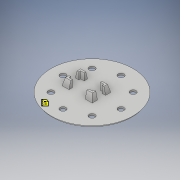
# Autodesk Inventor part: bottom_platform
Saved by Autodesk Inventor 2018 (Build 220112000, 112)
## iProperties
Created: 2018-04-16
Part Number: bottom_platform
Material: Generic
Document SubType Name: Modeling
Designer: scwu
Density: 1 g/cm^3
Appearance: Default
Author: scwu
Autodesk Inventor part; units mm, degrees
sketch "Sketch1" plane through (0, 0, 0) normal (0, 0, 1) x (1, 0, 0)
  arc A0 (68.484, -50.5) -> (70.5979, -47.5) centre (0, 0) ccw
  line L0 (0, -47.5) -> (70.5979, -47.5)
  line L1 (0, -47.5) -> (0, -50.5)
  line L2 (0, -50.5) -> (68.484, -50.5)
  dimension "d0" = 170.18
  dimension "d1" = 37.59
  dimension "d13" = 3
  constraints: 6 end point, 2 horizontal, 2 point on circle, 1 centre point, 1 coincident
  measures "d0" diameter of A0
  measures "d1" distance edge to line of A0 L0
  measures "d13" distance between parallel lines of L2 L0
revolve "Revolution1" add sketch "Sketch1" angle 360 about axis through (0, -47.5, 0) along (0, -1, 0)
ref_plane "Work Plane1" through (0, -35.5, 0) normal (0, 1, 0) x (1, 0, 0)
sketch "Sketch2" plane through (0, -35.5, 0) normal (0, 1, 0) x (1, 0, 0)
  line L0 (10.3, -10) -> (-29.7, -10) construction
  line L1 (-29.7, -10) -> (-29.7, 10) construction
  line L2 (-29.7, 10) -> (10.3, 10) construction
  line L3 (10.3, 10) -> (10.3, -10) construction
  line L4 (0, 0) -> (-20, 0) construction
  line L5 (10.3, 10) -> (10.3, 7)
  line L6 (10.3, 7) -> (13.3, 7)
  line L7 (13.3, 7) -> (13.3, 13)
  line L8 (13.3, 13) -> (4.3, 13)
  line L9 (4.3, 13) -> (4.3, 10)
  line L10 (10.3, 10) -> (4.3, 10)
  line L11 (-9.7, 10) -> (-9.7, -10) construction
  line L12 (-19.4, 0) -> (0.6, 0) construction
  line L13 (-29.7, 10) -> (-29.7, 7)
  line L14 (-29.7, 7) -> (-32.7, 7)
  line L15 (-32.7, 7) -> (-32.7, 13)
  line L16 (-32.7, 13) -> (-23.7, 13)
  line L17 (-23.7, 13) -> (-23.7, 10)
  line L18 (-29.7, 10) -> (-23.7, 10)
  line L19 (10.3, -10) -> (10.3, -7)
  line L20 (10.3, -7) -> (13.3, -7)
  line L21 (13.3, -7) -> (13.3, -13)
  line L22 (13.3, -13) -> (4.3, -13)
  line L23 (4.3, -13) -> (4.3, -10)
  line L24 (10.3, -10) -> (4.3, -10)
  line L25 (-29.7, -10) -> (-29.7, -7)
  line L26 (-23.7, -13) -> (-23.7, -10)
  line L27 (-32.7, -13) -> (-23.7, -13)
  line L28 (-29.7, -7) -> (-32.7, -7)
  line L29 (-32.7, -7) -> (-32.7, -13)
  line L30 (-29.7, -10) -> (-23.7, -10)
  dimension "d3" = 40
  dimension "d4" = 20
  dimension "d5" = 20
  dimension "d6" = 29.7
  dimension "d7" = 3
  dimension "d8" = 3
  dimension "d9" = 6
  dimension "d10" = 9
  constraints: 62 end point, 17 symmetric about line, 5 perpendicular, 2 horizontal, 2 midpoint, 2 parallel, 2 point on line, 1 collinear, 1 other
  measures "d3" distance of L1.end L2.end
  measures "d4" distance of L0.end L1.end
  measures "d5" distance of L4.start L4.end
  measures "d6" distance from line of L4.start L1
  measures "d7" distance of L2.end L5.end
  measures "d8" distance of L5.end L6.end
  measures "d9" distance of L6.end L7.end
  measures "d10" distance of L7.end L8.end
sketch "Sketch4" plane through (0, 0, 0) normal (0, 0, 1) x (1, 0, 0)
  arc A0 (0, -85.09) -> (85.09, 0) centre (0, 0) ccw
  line L0 (0, -85.09) -> (0, 0) construction
  line L1 (0, 0) -> (85.09, 0) construction
  dimension "d28" = 170.18
  constraints: 4 end point, 2 point on circle, 1 centre point, 1 coincident, 1 vertical
  measures "d28" diameter of A0
surface revolve "RevolutionSrf1" sketch "Sketch4" angle 360 about axis through (0, -85.09, 0) along (0, 1, 0) shown yes curves A0
sketch "Sketch5" plane through (0, -47.5, 0) normal (0, 1, 0) x (1, 0, 0)
  circle A0 centre (-50, 0) radius 5
  circle A1 centre (-35.3553, -35.3553) radius 5
  circle A2 centre (0, -50) radius 5
  circle A3 centre (35.3553, -35.3553) radius 5
  circle A4 centre (50, 0) radius 5
  circle A5 centre (35.3553, 35.3553) radius 5
  circle A6 centre (0, 50) radius 5
  circle A7 centre (-35.3553, 35.3553) radius 5
  point P0 (0, 0)
  dimension "d38" = 10
  dimension "d39" = 50
  dimension "d42" = 360
  constraints: 8 centre point, 17 other
  measures "d38" diameter of A0
  measures "d39" distance of A0.centre point (0, 0)
extrude "Extrusion3" cut sketch "Sketch5" against normal through all
sketch "Sketch6" plane through (0, -47.5, 0) normal (0, 1, 0) x (1, 0, 0)
  line L0 (-23.7, 10) -> (-29.7, 10)
  line L1 (-23.7, 10) -> (-23.7, 16)
  line L2 (-23.7, 16) -> (-35.7, 16)
  line L3 (-35.7, 16) -> (-35.7, 7)
  line L4 (-29.7, 7) -> (-29.7, 10)
  line L5 (-35.7, 7) -> (-29.7, 7)
  line L6 (-29.7, 7) -> (-29.7, 10)
  line L7 (-9.7, 10) -> (-9.7, -10) construction
  line L8 (-19.4, 0) -> (0.6, 0) construction
  point P0 (0, 0)
  dimension "d46" = 6
  dimension "d47" = 12
  dimension "d48" = 9
  dimension "d49" = 90
  constraints: 14 end point, 2 perpendicular, 1 collinear, 1 vertical
  measures "d46" distance of L0.start L1.end
  measures "d47" distance of L1.end L2.end
  measures "d48" distance of L2.end L3.end
  measures "d49" angle of L3 L2
sketch "Sketch7" plane through (0, -35.5, 0) normal (0, 1, 0) x (1, 0, 0)
  line L0 (-29.7, 10) -> (-23.7, 10)
  line L1 (-23.7, 10) -> (-23.7, 13)
  line L2 (-23.7, 13) -> (-32.7, 13)
  line L3 (-32.7, 13) -> (-32.7, 7)
  line L4 (-32.7, 7) -> (-29.7, 7)
  line L5 (-29.7, 7) -> (-29.7, 10)
  point P0 (0, 0)
  dimension "d51" = 6
  dimension "d52" = 3
  dimension "d53" = 90
  dimension "d54" = 9
  dimension "d55" = 90
  dimension "d56" = 6
  dimension "d57" = 3
  constraints: 12 end point, 4 perpendicular, 1 horizontal
  measures "d51" distance of L0.start L0.end
  measures "d52" distance of L0.end L1.end
  measures "d53" angle of L1 L0
  measures "d54" distance of L1.end L2.end
  measures "d55" angle of L2 L1
  measures "d56" distance of L2.end L3.end
  measures "d57" distance of L3.end L4.end
sketch "Sketch8" plane through (0, -35.5, 0) normal (0, 1, 0) x (1, 0, 0)
  point P0 (0, 0)
loft "Loft1" add profiles "Sketch6", "Sketch7"
ref_plane "Work Plane2" through (-9.7, -35.5, -10) normal (-1, 0, 0) x (0, 0, 1)
ref_plane "Work Plane3" through (-19.4, -35.5, 0) normal (0, 0, 1) x (1, 0, 0)
mirror "Mirror1" about plane through (-9.7, -35.5, -10) normal (-1, 0, 0) of "Loft1"
mirror "Mirror2" about plane through (-19.4, -35.5, 0) normal (0, 0, 1) of "Loft1", "Mirror1"
body "Solid1"
body "Srf1"
